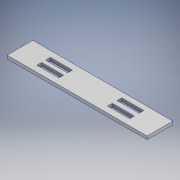
# Autodesk Inventor part: BK-BKT120-Front
Saved by Autodesk Inventor 2017 (Build 210142000, 142)
## iProperties
Created: 2016-09-24
Part Number: BK-BKT120-Front
Material: Aluminum 6061
Document SubType Name: Modeling
Designer: vslabsal
Density: 2.7 g/cm^3
Appearance: Aluminum - Flat
Author: vslabsal
Autodesk Inventor part; units mm, degrees
ref_plane "YZ Plane" through (0, 0, 0) normal (1, 0, 0) x (0, 1, 0)
ref_plane "XZ Plane" through (0, 0, 0) normal (0, 1, 0) x (-1, 0, 0)
ref_plane "XY Plane" through (0, 0, 0) normal (0, 0, 1) x (1, 0, 0)
sketch "Sketch1" plane through (0, 0, 0) normal (0, 0, 1) x (1, 0, 0)
  line L0 (-207.01, -38.1) -> (207.01, -38.1)
  line L1 (207.01, -38.1) -> (207.01, 38.1)
  line L2 (207.01, 38.1) -> (-207.01, 38.1)
  line L3 (-207.01, 38.1) -> (-207.01, -38.1)
  line L4 (-207.01, -38.1) -> (207.01, 38.1) construction
  line L5 (207.01, -38.1) -> (-207.01, 38.1) construction
  line L6 (72, -6) -> (137, -6)
  line L7 (137, -6) -> (137, -20)
  line L8 (137, -20) -> (72, -20)
  line L9 (72, -20) -> (72, -6)
  line L10 (72, -6) -> (137, -20) construction
  line L11 (137, -6) -> (72, -20) construction
  line L12 (-137, -6) -> (-72, -6)
  line L13 (-72, -6) -> (-72, -20)
  line L14 (-72, -20) -> (-137, -20)
  line L15 (-137, -20) -> (-137, -6)
  line L16 (-137, -6) -> (-72, -20) construction
  line L17 (-72, -6) -> (-137, -20) construction
  line L18 (-137, 20) -> (-72, 20)
  line L19 (-72, 20) -> (-72, 6)
  line L20 (-72, 6) -> (-137, 6)
  line L21 (-137, 6) -> (-137, 20)
  line L22 (-137, 20) -> (-72, 6) construction
  line L23 (-72, 20) -> (-137, 6) construction
  line L24 (72, 22) -> (137, 22)
  line L25 (137, 22) -> (137, 8)
  line L26 (137, 8) -> (72, 8)
  line L27 (72, 8) -> (72, 22)
  line L28 (72, 22) -> (137, 8) construction
  line L29 (137, 22) -> (72, 8) construction
  point P0 (0, 0)
  point P1 (0, 0)
  point P2 (104.5, -13)
  point P3 (-104.5, -13)
  point P4 (-104.5, 13)
  point P5 (104.5, 15)
  dimension "d0" = 414.02
  dimension "d1" = 76.2
  dimension "d2" = 65
  dimension "d3" = 14
  dimension "d4" = 65
  dimension "d5" = 14
  dimension "d6" = 65
  dimension "d7" = 14
  dimension "d8" = 65
  dimension "d9" = 14
  constraints: 60 end point, 10 midpoint, 10 parallel, 5 horizontal, 5 perpendicular
  measures "d0" distance of L0.start L0.end
  measures "d1" distance of L0.end L1.end
  measures "d2" distance of L7.end L8.end
  measures "d3" distance of L6.end L7.end
  measures "d4" distance of L13.end L14.end
  measures "d5" distance of L12.end L13.end
  measures "d6" distance of L19.end L20.end
  measures "d7" distance of L19.start L19.end
  measures "d8" distance of L26.start L27.start
  measures "d9" distance of L24.end L26.start
extrude "Extrusion1" add sketch "Sketch1" along normal blind 9.525
body "Solid1"
